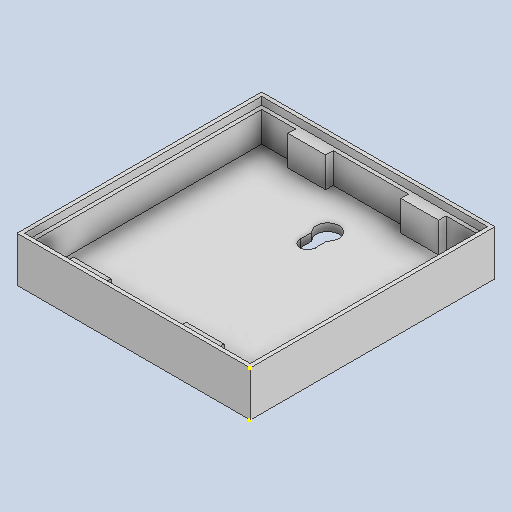
# Autodesk Inventor part: Shell 1
Saved by Autodesk Inventor 2022 (Build 260153000, 153)
## iProperties
Created: 2021-10-12
Part Number: Shell 1
Material: Generic
Document SubType Name: Modeling
Designer: Elisabeth
Density: 1 g/cm^3
Appearance: Default
Author: Elisabeth
Autodesk Inventor part; units mm, degrees
ref_plane "YZ Plane" through (0, 0, 0) normal (1, 0, 0) x (0, 1, 0)
ref_plane "XZ Plane" through (0, 0, 0) normal (0, 1, 0) x (-1, 0, 0)
ref_plane "XY Plane" through (0, 0, 0) normal (0, 0, 1) x (1, 0, 0)
sketch "Sketch1" plane through (0, 0, 0) normal (0, 1, 0) x (-1, 0, 0)
  point P0 (0, 0)
sketch "Sketch2" plane through (0, 0, 0) normal (0, 1, 0) x (-1, 0, 0)
  line L0 (0, 0) -> (62, 0)
  line L1 (62, 0) -> (62, -65)
  line L2 (62, -65) -> (0, -65)
  line L3 (0, -65) -> (0, 0)
  dimension "d0" = 62
  dimension "d1" = 65
  constraints: 8 end point, 2 parallel, 1 horizontal, 1 perpendicular
  measures "d0" distance of L1.end L2.end
  measures "d1" distance of L0.end L1.end
extrude "Extrusion1" add sketch "Sketch2" along normal blind 12
sketch "Sketch3" plane through (0, 12, 0) normal (0, 1, 0) x (1, 0, 0)
  point P0 (0, 0)
sketch "Sketch4" plane through (0, 12, 0) normal (0, 1, 0) x (1, 0, 0)
  line L0 (0, 65) -> (-62, 65) projected
  line L1 (-30.4814, 65) -> (-28.4814, 65)
  line L2 (-28.4814, 65) -> (-28.4814, 63)
  line L3 (-62, 65) -> (-62, 0) projected
  line L4 (-62, 36.8423) -> (-62, 38.8423)
  line L5 (-62, 38.8423) -> (-60, 38.8423)
  line L6 (-62, 0) -> (0, 0) projected
  line L7 (-28.4814, 0) -> (-30.4814, 0)
  line L8 (-30.4814, 0) -> (-30.4814, 2)
  line L9 (0, 0) -> (0, 65) projected
  line L10 (0, 38.8423) -> (0, 36.8423)
  line L11 (0, 36.8423) -> (-2, 36.8423)
  line L12 (-60, 63) -> (-2, 63)
  line L13 (-2, 63) -> (-2, 2)
  line L14 (-2, 2) -> (-60, 2)
  line L15 (-60, 2) -> (-60, 63)
  dimension "d5" = 2
  dimension "d6" = 2
  dimension "d7" = 2
  dimension "d8" = 2
  dimension "d9" = 2
  dimension "d10" = 2
  dimension "d11" = 2
  dimension "d12" = 2
  constraints: 24 end point, 8 point on line, 5 perpendicular, 2 parallel, 1 horizontal
  measures "d5" distance of L1.start L1.end
  measures "d6" distance of L1.end L2.end
  measures "d7" distance of L4.start L4.end
  measures "d8" distance of L4.end L5.end
  measures "d9" distance of L7.start L7.end
  measures "d10" distance of L7.end L8.end
  measures "d11" distance of L10.start L10.end
  measures "d12" distance of L10.end L11.end
extrude "Extrusion2" cut sketch "Sketch4" against normal blind 10 contours L12 L13 L14 L15
sketch "Sketch10" plane through (0, 2, 0) normal (0, 1, 0) x (1, 0, 0)
  line L0 (-2, 2) -> (-60, 2) projected
  line L1 (-31, 2) -> (-41, 2)
  line L2 (-41, 2) -> (-41, 4)
  line L3 (-41, 2) -> (-51, 2)
  line L4 (-51, 2) -> (-51, 4)
  line L5 (-51, 4) -> (-41, 4)
  line L6 (-41, 4) -> (-41, 2)
  line L7 (-60, 63) -> (-2, 63) projected
  line L8 (-51, 63) -> (-41, 63)
  line L9 (-41, 63) -> (-41, 61)
  line L10 (-41, 61) -> (-51, 61)
  line L11 (-51, 61) -> (-51, 63)
  line L12 (-60, 2) -> (-60, 63) projected
  line L13 (-21, 63) -> (-11, 63)
  line L14 (-11, 63) -> (-11, 61)
  line L15 (-11, 61) -> (-21, 61)
  line L16 (-21, 61) -> (-21, 63)
  line L17 (-21, 2) -> (-11, 2)
  line L18 (-11, 2) -> (-11, 4)
  line L19 (-11, 4) -> (-21, 4)
  line L20 (-21, 4) -> (-21, 2)
  line L21 (-2, 63) -> (-2, 2) projected
  point P0 (0, 0)
  dimension "d55" = 2
  dimension "d56" = 10
  dimension "d57" = 10
  dimension "d58" = 2
  dimension "d59" = 9
  dimension "d60" = 10
  dimension "d61" = 10
  dimension "d62" = 9
  dimension "d63" = 9
  constraints: 36 end point, 8 parallel, 5 horizontal, 5 perpendicular, 3 point on line
  measures "d55" distance of L1.end L2.end
  measures "d56" distance of L4.end L5.end
  measures "d57" distance of L9.end L10.end
  measures "d58" distance of L8.end L9.end
  measures "d59" distance between parallel lines of L12 L11
  measures "d60" distance of L14.end L15.end
  measures "d61" distance of L19.end L18.end
  measures "d62" distance between parallel lines of L21 L14
  measures "d63" distance between parallel lines of L21 L18
extrude "Extrusion5" add sketch "Sketch10" along normal blind 9 contours L0 L20 L19 L18 | L14 L15 L16 L7 | L0 L4 L5 L2 | L9 L10 L11 L7
sketch "Sketch12" plane through (0, 0, 0) normal (0, -1, 0) x (1, 0, 0)
  line L0 (0, 0) -> (0, -65) projected
  arc A0 (-33, -49.3087) -> (-29, -49.3087) centre (-31, -51.5448) ccw
  arc A1 (-29, -46.2034) -> (-33, -46.2034) centre (-31, -46.2034) ccw
  line L1 (-29, -46.2034) -> (-29, -49.3087)
  line L2 (-33, -46.2034) -> (-33, -49.3087)
  constraints: 4 end point, 4 point on circle, 2 centre point, 1 vertical
extrude "Extrusion7" cut sketch "Sketch12" against normal blind 10
sketch "Sketch13" plane through (0, 12, 0) normal (0, 1, 0) x (1, 0, 0)
  line L0 (-60, 2) -> (-60, 63) projected
  line L1 (-60, 4.6965) -> (-61, 4.6965)
  line L2 (-62, 65) -> (-62, 0) projected
  line L3 (-55.851, 2) -> (-55.851, 1)
  line L4 (-2, 63) -> (-2, 2) projected
  line L5 (-2, 53.5974) -> (-2, 54.5974)
  line L6 (-2, 54.5974) -> (-1, 54.5974)
  line L7 (0, 0) -> (0, 65) projected
  line L8 (-60, 63) -> (-2, 63) projected
  line L9 (-54.9589, 63) -> (-55.9589, 63)
  line L10 (-55.9589, 63) -> (-56.9589, 63)
  line L11 (-56.9589, 63) -> (-56.9589, 64)
  line L12 (-61, 1) -> (-1, 1)
  line L13 (-1, 1) -> (-1, 64)
  line L14 (-1, 64) -> (-61, 64)
  line L15 (-61, 64) -> (-61, 1)
  dimension "d81" = 1
  dimension "d82" = 1
  dimension "d83" = 1
  dimension "d84" = 1
  dimension "d85" = 1
  dimension "d86" = 1
  dimension "d87" = 1
  constraints: 22 end point, 6 point on line, 4 perpendicular, 2 parallel, 1 horizontal, 1 vertical
  measures "d81" distance of L1.start L1.end
  measures "d82" distance of L3.start L3.end
  measures "d83" distance of L5.start L5.end
  measures "d84" distance of L5.end L6.end
  measures "d85" distance of L9.start L9.end
  measures "d86" distance of L9.end L10.end
  measures "d87" distance of L10.end L11.end
extrude "Extrusion8" cut sketch "Sketch13" against normal blind 2
body "Solid1"
